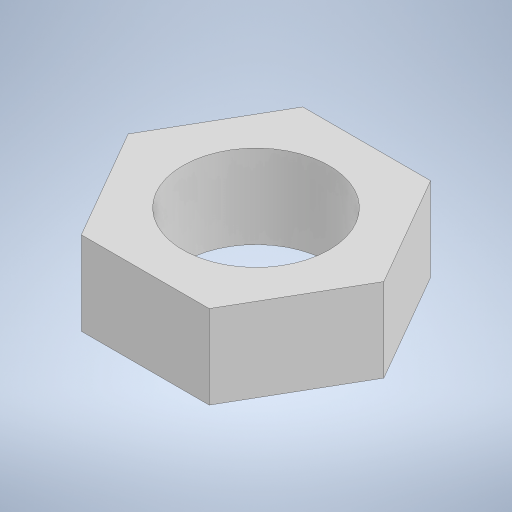
# Autodesk Inventor part: Nut
Saved by Autodesk Inventor 2024 (Build 280153000, 153)
## iProperties
Created: 2024-04-25
Part Number: Nut
Material: Generic
Document SubType Name: Modeling
Designer: auror
Density: 1 g/cm^3
Appearance: Default
Author: auror
Autodesk Inventor part; units mm, degrees
ref_plane "YZ Plane" through (0, 0, 0) normal (1, 0, 0) x (0, 1, 0)
ref_plane "XZ Plane" through (0, 0, 0) normal (0, 1, 0) x (-1, 0, 0)
ref_plane "XY Plane" through (0, 0, 0) normal (0, 0, 1) x (1, 0, 0)
sketch "Sketch1" plane through (0, 0, 0) normal (0, 1, 0) x (-1, 0, 0)
  line L0 (1.53, 2.65) -> (3.06, 0)
  line L1 (3.06, 0) -> (1.53, -2.65)
  line L2 (1.53, -2.65) -> (-1.53, -2.65)
  line L3 (-1.53, -2.65) -> (-3.0601, 0)
  line L4 (-3.0601, 0) -> (-1.53, 2.65)
  line L5 (-1.53, 2.65) -> (1.53, 2.65)
  circle A0 centre (0, 0) radius 1.75
  point P0 (-4.9823, -6.7157)
  point P1 (-7.6323, -6.7157)
  point P2 (-8.4592, -9.3657)
  point P3 (-7.6323, -12.0157)
  point P4 (-4.9823, -12.0157)
  point P5 (-3.1592, -9.3657)
  point P6 (-1.53, 2.65)
  dimension "d0" = 0
  dimension "d1" = 0
  dimension "d2" = 0
  dimension "d3" = 0
  dimension "d4" = 0
  dimension "d5" = 5.3
  dimension "d6" = 2.65
  dimension "d7" = 5.3
  dimension "d8" = 2.65
  dimension "d10" = 5.3
  dimension "d11" = 2.65
  dimension "d12" = 0
  dimension "d13" = 0
  dimension "d14" = 5.3
  dimension "d15" = 2.65
  dimension "d17" = 3.06
  dimension "d18" = 3.06
  dimension "d19" = 3.06
  dimension "d20" = 3.06
  dimension "d21" = 3.06
  dimension "d22" = 1.53
  dimension "d23" = 3.5
  constraints: 12 end point, 1 centre point, 1 coincident, 1 parallel
  measures "d0" vertical distance of point (-8.459, -9.366) point (-3.159, -9.366)
  measures "d1" horizontal distance of point (-7.632, -12.016) point (-7.632, -6.716)
  measures "d2" horizontal distance of point (-4.982, -12.016) point (-4.982, -6.716)
  measures "d3" vertical distance of point (-7.632, -6.716) point (-4.982, -6.716)
  measures "d4" vertical distance of point (-7.632, -12.016) point (-4.982, -12.016)
  measures "d5" distance of point (-4.982, -12.016) point (-4.982, -6.716)
  measures "d6" distance of point (-7.632, -6.716) point (-4.982, -6.716)
  measures "d7" distance of point (-3.159, -9.366) point (-8.459, -9.366)
  measures "d8" vertical distance of point (-4.982, -6.716) point (-3.159, -9.366)
  measures "d10" distance of L1.end L0.start
  measures "d11" vertical distance of point (0, 0) L0.start
  measures "d12" horizontal distance of L1.end L0.start
  measures "d13" horizontal distance of L2.end point (-1.53, 2.65)
  measures "d14" distance of point (-1.53, 2.65) L2.end
  measures "d15" vertical distance of point (0, 0) point (-1.53, 2.65)
  measures "d17" distance of L0.start L0.end
  measures "d18" distance of L1.end L0.end
  measures "d19" distance of L3.end point (-1.53, 2.65)
  measures "d20" distance of L3.end L2.end
  measures "d21" distance of point (-1.53, 2.65) L0.start
  measures "d22" horizontal distance of L0.start point (0, 0)
  measures "d23" diameter of A0
extrude "Extrusion1" add sketch "Sketch1" along normal blind 2
body "Solid1"
